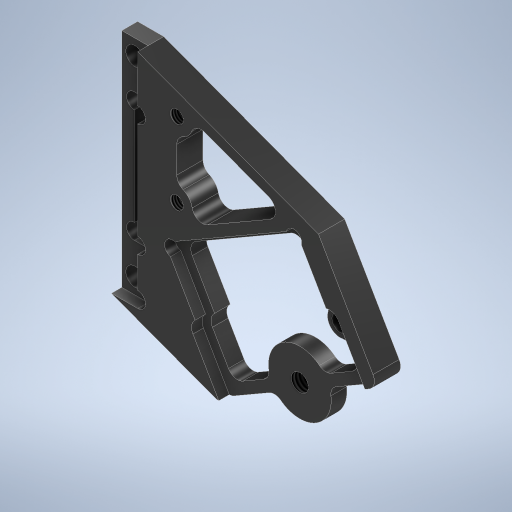
# Autodesk Inventor part: ShoulderIdlerSideFrame
Saved by Autodesk Inventor 2024.2 (Build 282272000, 272)
## iProperties
Created: 2024-01-17
Part Number: ShoulderIdlerSideFrame
Material: Aluminum 7075
Document SubType Name: Modeling
Designer: Masato Kubotera
Density: 2.81 g/cm^3
Appearance: Glossy - Black
Mass: 11.3574 g
Surface Area: 37.9697 cm^2
Volume: 4.04178 cm^3
Vendor: meviy
Author: Masato Kubotera
Autodesk Inventor part; units mm, degrees
ref_plane "YZ Plane" through (0, 0, 0) normal (1, 0, 0) x (0, 1, 0)
ref_plane "XZ Plane" through (0, 0, 0) normal (0, 1, 0) x (-1, 0, 0)
ref_plane "XY Plane" through (0, 0, 0) normal (0, 0, 1) x (1, 0, 0)
derived "ShoulderSideFrameBasis.ipt"
sketch "Sketch1" plane through (0, 0, 0) normal (1, 0, 0) x (0, 1, 0)
  line L0 (-1.5, 16.25) -> (-1.5, -26.25)
  line L1 (-1.5, 16.25) -> (3.5, 16.25)
  line L2 (3.5, 16.25) -> (3.5, -26.25)
  line L3 (3.5, -26.25) -> (-1.5, -26.25)
  line L4 (3.5, -26.25) -> (3.5, -28.1162)
  line L5 (13.1436, -23.4737) -> (40.8564, -7.4737)
  line L6 (40.8564, -7.4737) -> (62.3564, -44.7128) construction
  line L7 (62.3564, -44.7128) -> (34.6436, -60.7128) construction
  line L8 (34.6436, -60.7128) -> (13.1436, -23.4737) construction
  line L9 (13.1436, -23.4737) -> (62.3564, -44.7128) construction
  line L10 (40.8564, -7.4737) -> (34.6436, -60.7128) construction
  line L11 (16.8087, -24.8218) -> (40.1913, -11.3218) construction
  line L12 (40.1913, -11.3218) -> (53.6913, -34.7045) construction
  line L13 (53.6913, -34.7045) -> (30.3087, -48.2045) construction
  line L14 (30.3087, -48.2045) -> (16.8087, -24.8218) construction
  line L15 (16.8087, -24.8218) -> (53.6913, -34.7045) construction
  line L16 (40.1913, -11.3218) -> (30.3087, -48.2045) construction
  line L17 (27, -15.4737) -> (48.5, -52.7128) construction
  circle A0 centre (42.5, -42.3205) radius 8 construction
  line L18 (38.0742, 3.3452) -> (49.4898, -16.4272)
  line L19 (14.5292, -22.6737) -> (8.7792, -12.7144) construction
  line L20 (8.7792, -12.7144) -> (33.7208, 1.6856) construction
  line L21 (33.7208, 1.6856) -> (39.4708, -8.2737) construction
  arc A1 (57.6652, -47.4213) -> (56.3564, -34.3205) centre (42.5, -42.3205) ccw construction
  arc A2 (28.6436, -50.3205) -> (39.3348, -58.0043) centre (42.5, -42.3205) ccw construction
  line L22 (39.5141, -8.2487) -> (33.7391, 1.7539)
  line L23 (3.5, 16.25) -> (38.0742, 3.3452)
  line L24 (33.7391, 1.7539) -> (8.7109, -12.6961)
  line L25 (8.7109, -12.6961) -> (14.4859, -22.6987)
  arc A3 (34.7997, -0.0832) -> (31.9019, 0.6932) centre (33.3508, 0.305) ccw
  arc A4 (10.5481, -11.6355) -> (9.7716, -14.5332) centre (10.1598, -13.0844) ccw
  line L26 (1, 7.25) -> (3.5, 7.25) construction
  line L27 (3.5, 7.25) -> (3.5, -17.25) construction
  line L28 (3.5, -17.25) -> (1, -17.25) construction
  line L29 (1, -17.25) -> (1, 7.25) construction
  line L30 (1, 7.25) -> (3.5, -17.25) construction
  line L31 (3.5, 7.25) -> (1, -17.25) construction
  line L32 (1, -5) -> (3.5, -5) construction
  line L33 (2.25, 7.25) -> (2.25, -17.25) construction
  line L34 (3.5, 7.3) -> (0.9, 7.3)
  line L35 (0.9, 7.3) -> (0.9, -17.3)
  line L36 (0.9, -17.3) -> (3.5, -17.3)
  arc A5 (0.9, 7.3) -> (0.9, 4.3) centre (0.9, 5.8) ccw
  arc A6 (3.5, 4.3) -> (3.5, 7.3) centre (3.5, 5.8) ccw
  arc A7 (0.9, -14.3) -> (0.9, -17.3) centre (0.9, -15.8) ccw
  arc A8 (3.5, -17.3) -> (3.5, -14.3) centre (3.5, -15.8) ccw
  arc A9 (3.5, -26.25) -> (3.5, -23.25) centre (3.5, -24.75) ccw
  line L37 (1, 13.25) -> (1, -23.25) construction
  line L38 (13.1003, -23.4987) -> (19.1356, -33.9522)
  circle A10 centre (11, 9.25) radius 6 construction
  circle A11 centre (11, -5) radius 6 construction
  circle A12 centre (11, 9.25) radius 3 construction
  circle A13 centre (11, -5) radius 3 construction
  line L39 (11, 9.25) -> (11, -5) construction
  circle A14 centre (1, 13.25) radius 2.75 construction
  line L40 (11, 2.125) -> (3.5, 2.125) construction
  circle A15 centre (32.5, -25) radius 6
  line L41 (19.1356, -33.9522) -> (49.4898, -16.4272)
  line L42 (-1.5, -26.25) -> (19.2092, -33.9797)
  line L43 (40.8997, -7.4487) -> (46.935, -17.9022)
  line L44 (13.1003, -23.4987) -> (40.8997, -7.4487)
  line L45 (14.8323, -22.4987) -> (19.8677, -31.2202)
  line L46 (19.8677, -31.2202) -> (26.9019, -27.159)
  line L47 (44.203, -17.1702) -> (37.1688, -21.2314)
  line L48 (41.8357, -13.0699) -> (44.203, -17.1702)
  arc A16 (38.203, -9.9778) -> (41.8357, -13.0699) centre (40.1913, -11.3218) ccw
  line L49 (13.8243, 10.2617) -> (32.5009, 3.2907)
  line L50 (32.5009, 3.2907) -> (16.8962, -5.7187)
  arc A17 (11, 6.25) -> (13.8243, 10.2617) centre (11, 9.25) ccw
  arc A18 (13.9377, -4.392) -> (11, -2) centre (11, -5) ccw
  line L51 (11, 6.25) -> (11, -2)
  arc A19 (13.9377, -4.392) -> (16.8962, -5.7187) centre (15.8962, -3.9866) ccw
  line L52 (16.218, -21.6987) -> (10.943, -12.5622)
  line L53 (10.943, -12.5622) -> (32.507, -0.1122)
  line L54 (32.507, -0.1122) -> (38.203, -9.9778)
  point P0 (0, 0)
  point P1 (37.75, -34.0933)
  point P2 (35.25, -29.7631)
  point P3 (37.75, -34.0933)
  point P4 (14.4859, -22.6987)
  point P5 (2.25, -5)
  point P6 (0.9, -14.3)
  point P7 (3.5, -14.3)
  point P8 (10.5481, -11.6355)
  point P9 (8.7109, -12.6961)
  point P10 (8.7109, -12.6961)
  point P11 (9.7716, -14.5332)
  point P12 (27.9226, -28.8791)
  point P13 (38.1481, -22.9754)
  point P14 (46.935, -17.9022)
  point P15 (40.8564, -7.4737)
  point P16 (37.1688, -21.2314)
  point P17 (14.8323, -22.4987)
extrude "Extrusion1" add sketch "Sketch1" against normal blind 5 contours L1 L2 L34 A5 L35 A7 L36 L3 L0 | L3 L4 L42 | L23 L18 L41 L43 L44 L5 L22 A3 L24 A4 L25 L38 L42 L4 A9 L2 A8 A6 | L2 A9 | L38 L44 L5 L45 L46 A15 L41 | L41 A15 | A15 L41 | L41 A15 L47 L48 A16 L54 L5 L44 L43 | L25 L24 L22 L5 L54 L53 L52 | A4 L25 | A4 L24 | L22 A3 | L24 A3
extrude "Extrusion2" cut sketch "Sketch1" against normal blind 2 contours L1 L2 L34 A5 L35 A7 L36 L3 L0 | L2 A9 | L38 L44 L5 L45 L46 A15 L41 | L41 A15 | A15 L41 | L41 A15 L47 L48 A16 L54 L5 L44 L43 | L46 L45 L5 L54 A16 L48 L47 A15 | L25 L24 L22 L5 L54 L53 L52 | A4 L25 | L52 L53 L54 L5 | A4 L24 | L22 A3 | L24 A3
fillet "Inner-R2" radius 2 16 edges at (-1, 40.8997, -7.4487) (-2.5, 11, -2) (-2.5, 16.8962, -5.7187) (-2.5, 13.8243, 10.2617) (-2.5, 11, 6.25) (-2.5, 32.5009, 3.2907) (-3.5, 38.203, -9.9778) (-3.5, 41.8357, -13.0699) (-3.5, 44.203, -17.1702) (-3.5, 37.1688, -21.2314) (-3.5, 26.9019, -27.159) (-3.5, 19.8677, -31.2202) (-3.5, 10.943, -12.5622) (-3.5, 32.507, -0.1122) (-3.5, 14.8323, -22.4987) (-1, 13.1003, -23.4987)
fillet "Outer-R2" radius 2 4 edges at (-2.5, 49.4898, -16.4272) (-3.5, 38.1481, -22.9754) (-3.5, 27.9226, -28.8791) (-3.5, 19.1356, -33.9522)
hole "M4" at (0, 32.5, -25) direction (-1, 0, 0) diameter 3.242 end through all thread size "M4x0.7" class "6H" standard "ANSI Metric M Profile"
hole "Phi3.1" at (0, 40.1913, -11.3218) direction (-1, 0, 0) diameter 3.1 end through all
hole "Phi3.5" at (0, 1, 13.25) at (0, 1, -23.25) direction (-1, 0, 0) diameter 3.5 end through all
hole "M3" at (0, 11, 9.25) at (0, 11, -5) direction (-1, 0, 0) diameter 2.459 end through all thread size "M3x0.5" class "6H" standard "ANSI Metric M Profile"
body "Solid1"
